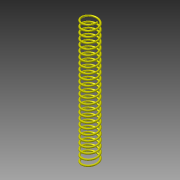
# Autodesk Inventor part: 知能ロボコンばね112038
Saved by Autodesk Inventor 2013 (Build 170138000, 138)
## iProperties
Created: 2014-05-12
Part Number: 知能ロボコンばね112038
Material: 一般
Document SubType Name: Modeling
Designer: horumo136
Density: 1 g/cm^3
Mass: 4.17484 g
Surface Area: 83.7563 cm^2
Volume: 4.17484 cm^3
Author: horumo136
Autodesk Inventor part; units mm, degrees
ref_plane "YZ Plane" through (0, 0, 0) normal (1, 0, 0) x (0, 1, 0)
sketch "スケッチ1" plane through (0, 0, 0) normal (0, 1, 0) x (-1, 0, 0)
  line L0 (0, 0) -> (-9, 0)
  line L1 (-9, 0) -> (-9, -10)
  line L2 (-9, 0) -> (-9, -150)
  dimension "d2" = 9
  dimension "d3" = 10
  dimension "d12" = 150
  constraints: 6 end point, 1 coincident, 1 collinear, 1 horizontal, 1 perpendicular
  measures "d2" distance of L0.start L0.end
  measures "d3" distance of L1.start L1.end
  measures "d12" distance of L1.start L2.end
sketch "スケッチ2" plane through (0, 0, 0) normal (0, 1, 0) x (-1, 0, 0)
  circle A0 centre (0, 0) radius 1
  point P0 (0, -1)
  point P1 (0, -1)
  dimension "d0" = 2
  constraints: 2 coincident, 1 vertical alignment, 2 other
coil "コイル1" sketch "スケッチ2" operation add axis through (9, 0, 0) along (0, 0, 1) pitch 6.383 turns 23.5 hand right
ref_plane "作業平面1" through (-1, 0, 0) normal (-1, 0, 0) x (0, -1, 0)
sketch "スケッチ3" plane through (-1, 0, 0) normal (-1, 0, 0) x (0, -1, 0)
  line L0 (0, 3.715) -> (0, -5.3018)
  point P0 (0, 0)
  constraints: 2 end point, 1 vertical
sketch "スケッチ4" plane through (0, 0, 0) normal (0, 1, 0) x (1, 0, 0)
  circle A0 centre (0, 0) radius 1 projected
  point P0 (-1, 0)
  point P1 (0, 1)
  constraints: 1 point on circle
ref_plane "作業平面2" through (0, 0, -1) normal (0, 0, -1) x (-1, 0, 0)
sketch "スケッチ5" plane through (0, 0, -1) normal (0, 0, -1) x (-1, 0, 0)
  line L0 (0, 0) -> (-9, 0)
  circle A0 centre (-9, 0) radius 9.0066
  constraints: 2 coincident, 2 end point, 1 centre point, 1 horizontal
ref_plane "作業平面3" through (9, 0, 0) normal (-1, 0, 0) x (0, -1, 0)
sketch "スケッチ6" plane through (9, 0, 0) normal (-1, 0, 0) x (0, -1, 0)
  line L0 (0, -1.0101) -> (0, 15.3766)
  point P0 (0, 0)
  constraints: 2 end point, 1 vertical
